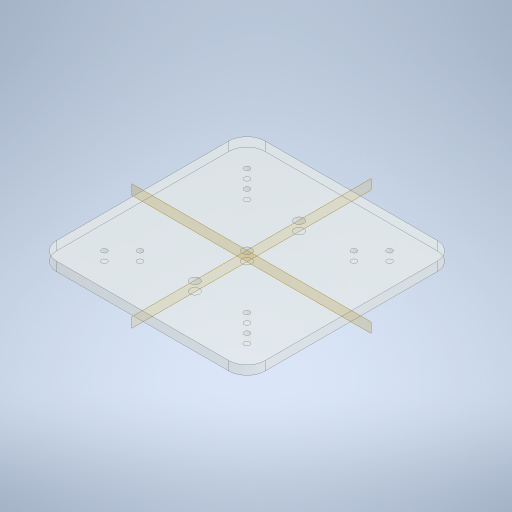
# Autodesk Inventor part: VESA adapter bracket
Saved by Autodesk Inventor 2023 (Build 270158000, 158)
## iProperties
Created: 2023-05-08
Part Number: VESA adapter bracket
Material: Generic
Document SubType Name: Modeling
Designer: rosam
Density: 1 g/cm^3
Appearance: Clear
Author: rosam
Autodesk Inventor part; units mm, degrees
ref_plane "YZ Plane" through (0, 0, 0) normal (1, 0, 0) x (0, 1, 0)
ref_plane "XZ Plane" through (0, 0, 0) normal (0, 1, 0) x (-1, 0, 0)
ref_plane "XY Plane" through (0, 0, 0) normal (0, 0, 1) x (1, 0, 0)
sketch "Sketch1" plane through (0, 0, 0) normal (0, 1, 0) x (-1, 0, 0)
  line L0 (60.325, 73.025) -> (-60.325, 73.025)
  line L1 (-73.025, 60.325) -> (-73.025, -60.325)
  line L2 (-60.325, -73.025) -> (60.325, -73.025)
  line L3 (73.025, -60.325) -> (73.025, 60.325)
  circle A0 centre (49.9999, 49.9999) radius 2
  circle A1 centre (49.9999, -49.9999) radius 2
  circle A2 centre (-49.9999, -49.9999) radius 2
  circle A3 centre (-49.9999, 49.9999) radius 2
  arc A4 (73.025, 60.325) -> (60.325, 73.025) centre (60.325, 60.325) ccw
  arc A5 (60.325, -73.025) -> (73.025, -60.325) centre (60.325, -60.325) ccw
  arc A6 (-60.325, 73.025) -> (-73.025, 60.325) centre (-60.325, 60.325) ccw
  arc A7 (-73.025, -60.325) -> (-60.325, -73.025) centre (-60.325, -60.325) ccw
  point P0 (0, 0)
  point P1 (73.025, 73.025)
  point P2 (-73.025, -73.025)
  point P3 (-73.025, 73.025)
  point P4 (73.025, -73.025)
  dimension "d0" = 73.025
  dimension "d1" = 73.025
  dimension "d2" = 146.05
  dimension "d3" = 146.05
  dimension "d4" = 4
  dimension "d5" = 4
  dimension "d6" = 4
  dimension "d7" = 4
  dimension "d8" = 99.9998
  dimension "d9" = 99.9998
  dimension "d10" = 99.9998
  dimension "d11" = 99.9998
  dimension "d12" = 23.0251
  dimension "d13" = 23.0251
  dimension "d14" = 23.0251
  dimension "d15" = 23.0251
  dimension "d16" = 23.0251
  dimension "d17" = 23.0251
  dimension "d18" = 23.0251
  dimension "d19" = 23.0251
  dimension "d40" = 12.7
  dimension "d41" = 12.7
  constraints: 8 centre point, 8 end point, 8 point on circle, 8 point on line, 8 tangent, 2 equal radius, 2 parallel, 1 horizontal, 1 perpendicular
  measures "d0" distance from line of point (0, 0) L3
  measures "d1" distance from line of point (0, 0) L0
  measures "d2" distance of point (73.025, 73.025) point (-73.025, 73.025)
  measures "d3" distance of point (-73.025, 73.025) point (-73.025, -73.025)
  measures "d4" diameter of A0
  measures "d5" diameter of A1
  measures "d6" diameter of A3
  measures "d7" diameter of A2
  measures "d8" distance of A1.centre A0.centre
  measures "d9" distance of A2.centre A3.centre
  measures "d10" distance of A0.centre A3.centre
  measures "d11" distance of A2.centre A1.centre
  measures "d12" distance from line of L3 A0.centre
  measures "d13" distance from line of L0 A0.centre
  measures "d14" distance from line of L2 A2.centre
  measures "d15" distance from line of L1 A2.centre
  measures "d16" distance from line of L2 A1.centre
  measures "d17" distance from line of L3 A1.centre
  measures "d18" distance from line of L0 A3.centre
  measures "d19" distance from line of L1 A3.centre
  measures "d40" radius of A4
  measures "d41" radius of A5
extrude "Extrusion1" add sketch "Sketch1" along normal blind 6.35
sketch "Sketch2" plane through (0, 6.35, 0) normal (0, 1, 0) x (1, 0, 0)
  circle A0 centre (-37.5, -37.5) radius 2
  circle A1 centre (-37.5, 37.5) radius 2
  circle A2 centre (37.5, -37.5) radius 2
  circle A3 centre (37.5, 37.5) radius 2
  line L0 (-60.325, -73.025) -> (60.325, -73.025) projected
  line L1 (-73.025, 60.325) -> (-73.025, -60.325) projected
  line L2 (73.025, -60.325) -> (73.025, 60.325) projected
  line L3 (60.325, 73.025) -> (-60.325, 73.025) projected
  point P0 (0, 0)
  point P1 (-76.2, -76.2)
  point P2 (76.2, -76.2)
  point P3 (-76.2, 76.2)
  point P4 (76.2, 76.2)
  point P5 (-60.325, 73.025)
  dimension "d22" = 4
  dimension "d23" = 4
  dimension "d24" = 4
  dimension "d25" = 4
  dimension "d26" = 75
  dimension "d27" = 75
  dimension "d28" = 75
  dimension "d29" = 75
  dimension "d30" = 35.525
  dimension "d31" = 35.525
  dimension "d32" = 35.525
  dimension "d33" = 35.525
  dimension "d34" = 35.525
  dimension "d35" = 35.525
  dimension "d36" = 35.525
  dimension "d37" = 35.525
  constraints: 4 centre point, 4 other
  measures "d22" diameter of A0
  measures "d23" diameter of A1
  measures "d24" diameter of A3
  measures "d25" diameter of A2
  measures "d26" distance of A1.centre A0.centre
  measures "d27" distance of A3.centre A2.centre
  measures "d28" distance of A0.centre A2.centre
  measures "d29" distance of A3.centre A1.centre
extrude "Extrusion2" cut sketch "Sketch2" against normal blind 6.35
sketch "Sketch3" plane through (0, 6.35, 0) normal (0, 1, 0) x (1, 0, 0)
  circle A0 centre (0, -36.5125) radius 3.302
  circle A1 centre (0, 0) radius 3.302
  circle A2 centre (0, 36.5125) radius 3.302
  line L0 (60.325, 73.025) -> (-60.325, 73.025) projected
  line L1 (-60.325, -73.025) -> (60.325, -73.025) projected
  line L2 (73.025, -60.325) -> (73.025, 60.325) projected
  line L3 (-73.025, 60.325) -> (-73.025, -60.325) projected
  point P0 (-73.025, 0)
  dimension "d52" = 6.604
  dimension "d53" = 6.604
  dimension "d54" = 6.604
  dimension "d61" = 36.5125
  dimension "d62" = 36.5125
  dimension "d63" = 36.5125
  dimension "d64" = 36.5125
  constraints: 3 centre point, 2 vertical alignment, 1 coincident, 1 midpoint
  measures "d52" diameter of A0
  measures "d53" diameter of A1
  measures "d54" diameter of A2
  measures "d61" distance of point (0, 0) A2.centre
  measures "d62" distance of A0.centre point (0, 0)
  measures "d63" distance from line of L0 A2.centre
  measures "d64" distance from line of L1 A0.centre
extrude "Extrusion3" cut sketch "Sketch3" against normal blind 6.35
ref_plane "Work Plane1" through (0, 0, 60.325) normal (1, 0, 0) x (0, 0, -1)
ref_plane "Work Plane2" through (-60.325, 0, 0) normal (0, 0, 1) x (1, 0, 0)
equation "\"d0\" = 0.5 * d2"
equation "\"d1\" = 0.5 * d3"
equation "\"d2\" = d3"
equation "\"d5\" = d4"
equation "\"d6\" = d4"
equation "\"d7\" = d4"
equation "\"d9\" = d8"
equation "\"d11\" = d10"
equation "\"d12\" = d17"
equation "\"d13\" = d16"
equation "\"d14\" = d13"
equation "\"d15\" = d12"
equation "\"d23\" = d22"
equation "\"d24\" = d22"
equation "\"d25\" = d22"
equation "\"d27\" = d26"
equation "\"d29\" = d28"
equation "\"d30\" = d36"
equation "\"d31\" = d37"
equation "\"d32\" = d31"
equation "\"d33\" = d30"
equation "\"d52\" = d53"
equation "\"d54\" = d53"
equation "\"d61\" = d63"
equation "\"d62\" = d64"
body "Solid1"
